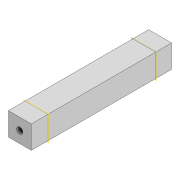
# Autodesk Inventor part: supports
Saved by Autodesk Inventor 2020 (Build 240168000, 168)
## iProperties
Created: 2019-11-23
Part Number: supports
Material: Generic
Document SubType Name: Modeling
Designer: ball
Density: 1 g/cm^3
Appearance: Default
Author: ball
Autodesk Inventor part; units mm, degrees
ref_plane "YZ Plane" through (0, 0, 0) normal (1, 0, 0) x (0, 1, 0)
ref_plane "XZ Plane" through (0, 0, 0) normal (0, 1, 0) x (-1, 0, 0)
ref_plane "XY Plane" through (0, 0, 0) normal (0, 0, 1) x (1, 0, 0)
ref_plane "Work Plane1" through (0, 0, 0) normal (0, 0, 1) x (1, 0, 0)
sketch "Sketch1" plane through (0, 0, 0) normal (0, 0, 1) x (1, 0, 0)
  circle A0 centre (-5.3931, -215.9272) radius 1.778 construction
  line L0 (0.9569, -209.5772) -> (-11.7431, -209.5772)
  line L1 (-11.7431, -209.5772) -> (-11.7431, -222.2772)
  line L2 (-11.7431, -222.2772) -> (0.9569, -222.2772)
  line L3 (0.9569, -222.2772) -> (0.9569, -209.5772)
  line L4 (0.9569, -209.5772) -> (-11.7431, -222.2772) construction
  line L5 (-11.7431, -209.5772) -> (0.9569, -222.2772) construction
  circle A1 centre (-5.3931, -215.9272) radius 1.7
  point P0 (0, 0)
  dimension "d0" = 12.7
  dimension "d1" = 12.7
  dimension "d2" = 3.4
  constraints: 12 end point, 2 midpoint, 2 parallel, 1 centre point, 1 coincident, 1 horizontal, 1 perpendicular
  measures "d0" distance of L2.end L1.end
  measures "d1" distance of L1.end L0.end
  measures "d2" diameter of A1
ref_plane "Work Plane2" through (-150.1545, -254.8124, 77.677) normal (0, 0, -1) x (0, 1, 0)
extrude "Extrusion1" add sketch "Sketch1" along normal up to surface (77.677 mm away)
ref_plane "Work Plane3" through (0, 0, 9) normal (0, 0, -1) x (-1, 0, 0)
sketch "Sketch2" plane through (0, 0, 9) normal (0, 0, -1) x (-1, 0, 0)
  circle A0 centre (5.3931, -215.9272) radius 1.7 construction
  circle A1 centre (5.3931, -215.9272) radius 3.45 construction
  line L0 (11.7431, -218.915) -> (3.6681, -218.915)
  line L1 (3.6681, -218.915) -> (1.9431, -215.9272)
  line L2 (1.9431, -215.9272) -> (3.6681, -212.9394)
  line L3 (3.6681, -212.9394) -> (11.7431, -212.9394)
  line L4 (11.7431, -212.9394) -> (11.7431, -218.915)
  line L5 (11.7431, -209.5772) -> (11.7431, -222.2772) projected
  line L6 (11.7431, -218.915) -> (3.6681, -218.915)
  line L7 (3.6681, -218.915) -> (1.9431, -215.9272)
  line L8 (1.9431, -215.9272) -> (3.6681, -212.9394)
  line L9 (3.6681, -212.9394) -> (11.7431, -212.9394)
  line L10 (11.7431, -212.9394) -> (11.7431, -218.915)
  point P0 (0, 0)
  dimension "d6" = 6.9
  constraints: 20 end point, 2 coincident, 1 centre point, 1 collinear, 6 other
  measures "d6" diameter of A1
extrude "Extrusion2" cut sketch "Sketch2" against normal blind 4.4
ref_plane "Work Plane4" through (-11.7431, -222.2772, 68.677) normal (0, 0, 1) x (1, 0, 0)
sketch "Sketch3" plane through (-11.7431, -222.2772, 68.677) normal (0, 0, 1) x (1, 0, 0)
  line L0 (0, 9.3378) -> (8.075, 9.3378)
  line L1 (8.075, 9.3378) -> (9.8, 6.35)
  line L2 (9.8, 6.35) -> (8.075, 3.3622)
  line L3 (8.075, 3.3622) -> (0, 3.3622)
  line L4 (0, 3.3622) -> (0, 9.3378)
  circle A0 centre (6.35, 6.35) radius 1.7 construction
  circle A1 centre (6.35, 6.35) radius 3.45 construction
  point P0 (11.7431, 222.2772)
  dimension "d10" = 6.9
  constraints: 10 end point, 1 centre point, 1 coincident
  measures "d10" diameter of A1
extrude "Extrusion3" cut sketch "Sketch3" against normal blind 4.4
body "Solid1"
